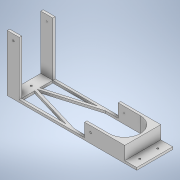
# Autodesk Inventor part: frame
Saved by Autodesk Inventor 2020 (Build 240168000, 168)
## iProperties
Created: 2020-02-27
Part Number: frame
Material: Типовые
Document SubType Name: Modeling
Designer: CSS38
Density: 1 g/cm^3
Appearance: По умолчанию
Author: CSS38
Autodesk Inventor part; units mm, degrees
ref_plane "YZ Plane" through (0, 0, 0) normal (1, 0, 0) x (0, 1, 0)
ref_plane "XZ Plane" through (0, 0, 0) normal (0, 1, 0) x (-1, 0, 0)
ref_plane "XY Plane" through (0, 0, 0) normal (0, 0, 1) x (1, 0, 0)
sketch "Эскиз1" plane through (0, 0, 0) normal (0, 1, 0) x (-1, 0, 0)
  line L0 (54, 15) -> (-54, 15)
  line L1 (-54, 15) -> (-54, -15)
  line L2 (-54, -15) -> (54, -15)
  line L3 (54, -15) -> (54, 15)
  line L4 (-54, 15) -> (54, -15) construction
  line L5 (-54, -15) -> (54, 15) construction
  line L6 (0, -21) -> (0, 21) construction
  line L7 (44, -13) -> (7.0585, -13)
  line L8 (-44, -13) -> (-44, 13)
  line L9 (-44, 13) -> (0, 13)
  line L10 (44, 13) -> (44, 2.0855)
  line L11 (75.6, 0) -> (-75.6, 0) construction
  line L12 (49, -15) -> (49, 15) construction
  line L13 (0, -13) -> (44, 0)
  line L14 (44, -2.0855) -> (7.0585, -13)
  line L15 (0, -15) -> (0, -13) construction
  line L16 (0, 13) -> (0, 15) construction
  line L17 (44, -2.0855) -> (43.4333, -0.1674) construction
  line L18 (44, 0) -> (0, 13)
  line L19 (44, 2.0855) -> (7.0585, 13)
  line L20 (44, 2.0855) -> (43.4333, 0.1674) construction
  line L21 (44, 2.0855) -> (44, -2.0855) construction
  line L22 (44, -2.0855) -> (44, -13)
  line L23 (7.0585, -13) -> (0, -13) construction
  line L24 (0, -13) -> (-44, -13)
  line L25 (7.0585, 13) -> (44, 13)
  line L26 (0, 13) -> (7.0585, 13) construction
  point P0 (0, 0)
  point P1 (0, -14)
  point P2 (0, 14)
  point P3 (0, 0)
  dimension "d0" = 108
  dimension "d8" = 10
  dimension "d9" = 5
  dimension "d28" = 26
  dimension "d46" = 2
  dimension "d47" = 10
  constraints: 50 end point, 16 parallel, 9 point on line, 7 midpoint, 7 perpendicular, 3 equal length, 2 vertical alignment, 1 horizontal
  measures "d0" distance of L2.end L1.end
  measures "d8" distance between parallel lines of L1 L8
  measures "d9" distance between parallel lines of L3 L12
  measures "d28" distance of L8.start L8.end
  measures "d46" distance of L15.start L13.start
  measures "d47" distance between parallel lines of L3 L10
extrude "Выдавливание1" add sketch "Эскиз1" along normal blind 2
sketch "Эскиз2" plane through (0, 0, 0) normal (0, 1, 0) x (-1, 0, 0)
  line L0 (-42, -13) -> (-42, 13) construction
  line L1 (-42, -13) -> (-29, -13) construction
  line L2 (-10.5, -13) -> (-10.5, -15)
  line L3 (-10.5, -15) -> (-44, -15)
  line L4 (-42, 13) -> (-29, 13) construction
  line L5 (-10.5, 15) -> (-44, 15)
  line L6 (-10.5, 13) -> (-10.5, 15)
  arc A0 (-29, 13) -> (-29, -13) centre (-29, 0) ccw
  line L7 (-29, -13) -> (-10.5, -13)
  line L8 (-29, 13) -> (-10.5, 13)
  line L9 (-44, -15) -> (-44, 15)
  line L10 (-44, -13) -> (-44, 13) construction
  line L11 (0, -13) -> (-44, -13) construction
  line L12 (-54, -15) -> (54, -15) construction
  line L13 (-44, 13) -> (0, 13) construction
  line L14 (54, 15) -> (-54, 15) construction
  point P0 (0, 0)
  dimension "d17" = 31.5
  dimension "d48" = 2
  constraints: 20 end point, 8 collinear, 3 tangent, 2 parallel, 2 point on circle, 2 vertical, 1 centre point, 1 horizontal, 1 perpendicular
  measures "d17" distance of L0.start L2.start
  measures "d48" distance between parallel lines of L9 L0
extrude "Выдавливание2" add sketch "Эскиз2" along normal blind 13
sketch "Эскиз4" plane through (0, 2, 0) normal (0, 1, 0) x (1, 0, 0)
  line L0 (-54, 15) -> (-54, -15) construction
  line L1 (-44, 13) -> (-54, 13)
  line L2 (-54, 13) -> (-54, 15)
  line L3 (-54, 15) -> (-44, 15)
  line L4 (-44, 15) -> (-44, 13)
  line L5 (44, -13) -> (0, -13) construction
  line L6 (-54, -15) -> (54, -15) construction
  line L7 (-44, -13) -> (-54, -13)
  line L8 (-54, -13) -> (-54, -15)
  line L9 (-54, -15) -> (-44, -15)
  line L10 (-44, -15) -> (-44, -13)
  point P0 (0, 0)
  point P1 (10.5, -13)
  point P2 (-44, -15)
  constraints: 16 end point, 4 parallel, 2 coincident, 2 horizontal, 2 perpendicular
extrude "Выдавливание4" add sketch "Эскиз4" along normal blind 45
sketch "Эскиз3" plane through (-54, 0, 15) normal (0, 0, 1) x (1, 0, 0)
  line L0 (64.5, 2) -> (64.5, 13) construction
  line L1 (64.5, 13) -> (74.5, 13) construction
  line L2 (74.5, 13) -> (74.5, 3) construction
  line L3 (74.5, 3) -> (64.5, 3) construction
  line L4 (64.5, 3) -> (64.5, 13) construction
  line L5 (64.5, 2) -> (54, 2) construction
  line L6 (74.5, 3) -> (64.5, 13) construction
  line L7 (74.5, 13) -> (64.5, 3) construction
  circle A0 centre (69.5, 8) radius 0.5
  line L8 (0, 47) -> (10, 47) construction
  line L9 (10, 2) -> (10, 47) construction
  line L10 (0, 47) -> (10, 47) construction
  line L11 (10, 47) -> (10, 37) construction
  line L12 (10, 37) -> (0, 37) construction
  line L13 (0, 37) -> (0, 47) construction
  line L14 (0, 37) -> (10, 47) construction
  line L15 (0, 0) -> (0, 47) construction
  line L16 (10, 37) -> (0, 47) construction
  circle A1 centre (5, 42) radius 0.5
  point P0 (54, 0)
  point P1 (128, 2)
  dimension "d20" = 10
  dimension "d21" = 1
  dimension "d26" = 10
  dimension "d27" = 1
  constraints: 24 end point, 4 parallel, 4 perpendicular, 2 centre point, 2 horizontal, 2 midpoint, 1 point on line, 1 other
  measures "d20" distance of L2.end L3.end
  measures "d21" diameter of A0
  measures "d26" distance of L10.end L11.end
  measures "d27" diameter of A1
hole "Отверстие1" at (-49, 42, 15) at (15.5, 8, 15) direction (0, 0, -1) diameter 1 depth 2 countersink diameter 1.5 countersink angle 90
mirror "Зеркальное отражение1" about plane through (0, 0, 0) normal (0, 0, 1) of "Отверстие1"
sketch "Эскиз5" plane through (0, 2, 0) normal (0, 1, 0) x (1, 0, 0)
  line L0 (10.5, 13) -> (10.5, 15) construction
  line L1 (-44, 15) -> (10.5, 15) construction
  line L2 (-54, 15) -> (-44, 15) construction
  line L3 (-54, 13) -> (-54, 15) construction
  line L4 (-44, 13) -> (-54, 13) construction
  line L5 (-44, -13) -> (-44, -15) construction
  line L6 (-44, -15) -> (-54, -15) construction
  line L7 (-54, -15) -> (-54, -13) construction
  line L8 (-54, -13) -> (-54, 13) construction
  line L9 (10.5, -15) -> (10.5, -13) construction
  line L10 (10.5, 15) -> (44, 15) construction
  line L11 (54, -15) -> (44, -15) construction
  line L12 (54, 15) -> (54, -15) construction
  line L13 (44, 15) -> (54, 15) construction
  line L14 (-44, 15) -> (-44, 13) construction
  line L15 (-54, -13) -> (-44, -13) construction
  line L16 (44, -15) -> (10.5, -15) construction
  line L17 (54, 15) -> (-54, 15) construction
  line L18 (54, 15) -> (44, 0) construction
  line L19 (-54, -15) -> (54, -15) construction
  line L20 (54, -15) -> (44, 0) construction
  line L21 (-54, 13) -> (-44, -13) construction
  line L22 (-44, -13) -> (-44, -2.0855) construction
  line L23 (-54, -13) -> (-44, 13) construction
  line L24 (54, -15) -> (54, 15) construction
  line L25 (54, 0) -> (44, 15) construction
  line L26 (44, -15) -> (54, 0) construction
  circle A0 centre (-49, 0) radius 0.5
  circle A1 centre (49, 7.5) radius 0.5
  circle A2 centre (49, -7.5) radius 0.5
  line L27 (-44, 2.0855) -> (-7.0585, 13) projected
  line L28 (-7.0585, 13) -> (-44, 13) projected
  line L29 (-44, -13) -> (-7.0585, -13) projected
  line L30 (-7.0585, -13) -> (-44, -2.0855) projected
  line L31 (-44, -2.0855) -> (-44, -13) projected
  line L32 (-44, 13) -> (-44, 2.0855) projected
  line L33 (10.5, 13) -> (0, 13) projected
  line L34 (0, 13) -> (-44, 0) projected
  line L35 (-44, 0) -> (0, -13) projected
  line L36 (0, -13) -> (10.5, -13) projected
  line L37 (10.5, -13) -> (29, -13) projected
  arc A3 (29, -13) -> (29, 13) centre (29, 0) ccw projected
  line L38 (29, 13) -> (10.5, 13) projected
  line L39 (44, 15) -> (44, -15) projected
  line L40 (10.5, -15) -> (-44, -15) projected
  point P0 (0, 0)
  dimension "d38" = 1
  constraints: 12 end point, 4 midpoint, 3 centre point, 2 equal radius
  measures "d38" diameter of A0
hole "Отверстие2" at (-49, 2, 0) at (49, 2, 7.5) at (49, 2, -7.5) direction (0, -1, 0) diameter 1 end through all countersink diameter 1.5 countersink angle 90
